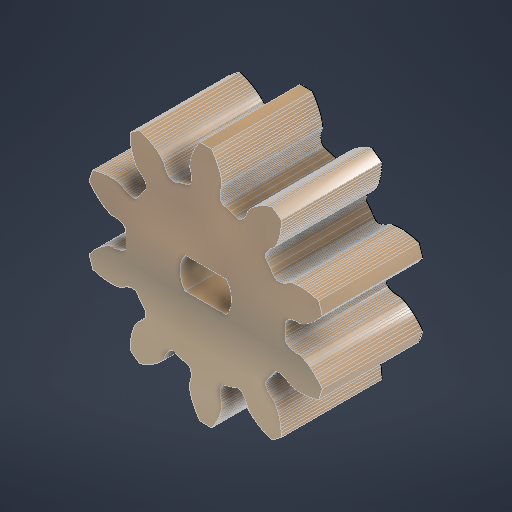
# Autodesk Inventor part: drive_gear_v1
Saved by Autodesk Inventor 2026.1 (Build 301233020, 233B)
## iProperties
Created: 2025-12-19
Part Number: drive_gear_v1
Material: Wood (Maple)
Document SubType Name: Modeling
Designer: colin
Density: 0.67 g/cm^3
Appearance: Natural Maple - Glossy Dark Tint
Autodesk Inventor part; units mm, degrees
(part 1 of 2)
ref_plane "YZ Plane" through (0, 0, 0) normal (1, 0, 0) x (0, 1, 0)
ref_plane "XZ Plane" through (0, 0, 0) normal (0, 1, 0) x (-1, 0, 0)
ref_plane "XY Plane" through (0, 0, 0) normal (0, 0, 1) x (1, 0, 0)
sketch "Sketch1" plane through (0, 0, 0) normal (0, 0, 1) x (1, 0, 0)
  point P0 (0, 0)
sketch "0" plane through (0, 0, 0) normal (0, 0, 1) x (1, 0, 0)
  line L0 (117.0437, 1.525) -> (112.9563, 1.525)
  line L1 (112.9563, -1.525) -> (117.0437, -1.525)
  line L2 (-25.3188, 0) -> (151.9129, 0) projected
  arc A0 (112.9563, 1.525) -> (112.9563, -1.525) centre (115, 0) ccw
  arc A1 (117.0437, -1.525) -> (117.0437, 1.525) centre (115, 0) ccw
  point P0 (119.0458, 0)
  point P1 (115.2341, -1.525)
  dimension "d8" = 3.05
  dimension "d9" = 2.55
  dimension "d10" = 2.55
  constraints: 4 end point, 4 point on circle, 2 centre point, 1 horizontal, 1 parallel, 1 point on line
  measures "d8" distance between parallel lines of L0 L1
  measures "d9" radius of A1
  measures "d10" radius of A0
sketch "layer0" plane through (0, 0, 0) normal (0, 0, 1) x (1, 0, 0)
  line L0 (107.4857, -9.0966) -> (107.5036, -8.8065)
  line L1 (107.5036, -8.8065) -> (107.532, -8.5336)
  line L2 (107.532, -8.5336) -> (107.5694, -8.2786)
  line L3 (107.5694, -8.2786) -> (107.6141, -8.0429)
  line L4 (107.6141, -8.0429) -> (107.6654, -7.8231)
  line L5 (107.6654, -7.8231) -> (107.721, -7.6228)
  line L6 (107.721, -7.6228) -> (107.7801, -7.4403)
  line L7 (107.7801, -7.4403) -> (107.8409, -7.2761)
  line L8 (107.8409, -7.2761) -> (107.9625, -7.0011)
  line L9 (107.9625, -7.0011) -> (108.0758, -6.7937)
  line L10 (108.0758, -6.7937) -> (108.1683, -6.6535)
  line L11 (108.1683, -6.6535) -> (108.218, -6.5889)
  line L12 (108.218, -6.5889) -> (108.3789, -6.4763)
  line L13 (108.3789, -6.4763) -> (108.5412, -6.345)
  line L14 (108.5412, -6.345) -> (108.681, -6.2122)
  line L15 (108.681, -6.2122) -> (108.7986, -6.0795)
  line L16 (108.7986, -6.0795) -> (108.8943, -5.9486)
  line L17 (108.8943, -5.9486) -> (108.9684, -5.821)
  line L18 (108.9684, -5.821) -> (109.0215, -5.6982)
  line L19 (109.0215, -5.6982) -> (109.054, -5.5819)
  line L20 (109.054, -5.5819) -> (109.0667, -5.4735)
  line L21 (109.0667, -5.4735) -> (109.0602, -5.3745)
  line L22 (109.0602, -5.3745) -> (109.0355, -5.2862)
  line L23 (109.0355, -5.2862) -> (108.987, -5.2014)
  line L24 (108.987, -5.2014) -> (108.8344, -5.0188)
  line L25 (108.8344, -5.0188) -> (108.5683, -4.6729)
  line L26 (108.5683, -4.6729) -> (108.3216, -4.313)
  line L27 (108.3216, -4.313) -> (108.1951, -4.1114)
  line L28 (108.1951, -4.1114) -> (108.1294, -4.0391)
  line L29 (108.1294, -4.0391) -> (108.0531, -3.9883)
  line L30 (108.0531, -3.9883) -> (107.9608, -3.9515)
  line L31 (107.9608, -3.9515) -> (107.8538, -3.9301)
  line L32 (107.8538, -3.9301) -> (107.7332, -3.9251)
  line L33 (107.7332, -3.9251) -> (107.6001, -3.9376)
  line L34 (107.6001, -3.9376) -> (107.4558, -3.9687)
  line L35 (107.4558, -3.9687) -> (107.3017, -4.0192)
  line L36 (107.3017, -4.0192) -> (107.1392, -4.0901)
  line L37 (107.1392, -4.0901) -> (106.9697, -4.182)
  line L38 (106.9697, -4.182) -> (106.7947, -4.2958)
  line L39 (106.7947, -4.2958) -> (106.6379, -4.414)
  line L40 (106.6379, -4.414) -> (106.561, -4.4413)
  line L41 (106.561, -4.4413) -> (106.3991, -4.4859)
  line L42 (106.3991, -4.4859) -> (106.1668, -4.5296)
  line L43 (106.1668, -4.5296) -> (105.8678, -4.5603)
  line L44 (105.8678, -4.5603) -> (105.6928, -4.5674)
  line L45 (105.6928, -4.5674) -> (105.5009, -4.5671)
  line L46 (105.5009, -4.5671) -> (105.2933, -4.5582)
  line L47 (105.2933, -4.5582) -> (105.0683, -4.539)
  line L48 (105.0683, -4.539) -> (104.8304, -4.5087)
  line L49 (104.8304, -4.5087) -> (104.5763, -4.4654)
  line L50 (104.5763, -4.4654) -> (104.308, -4.4081)
  line L51 (104.308, -4.4081) -> (104.0266, -4.3355)
  line L52 (104.0266, -4.3355) -> (103.7825, -4.2622)
  arc A0 (103.4196, -3.1453) -> (103.7825, -4.2622) centre (115.0001, 0) ccw
  line L53 (103.4196, -3.1453) -> (103.574, -2.9425)
  line L54 (103.574, -2.9425) -> (103.759, -2.7184)
  line L55 (103.759, -2.7184) -> (103.9423, -2.5143)
  line L56 (103.9423, -2.5143) -> (104.1225, -2.33)
  line L57 (104.1225, -2.33) -> (104.2971, -2.1655)
  line L58 (104.2971, -2.1655) -> (104.4678, -2.0178)
  line L59 (104.4678, -2.0178) -> (104.6306, -1.8885)
  line L60 (104.6306, -1.8885) -> (104.7857, -1.7756)
  line L61 (104.7857, -1.7756) -> (104.9314, -1.6785)
  line L62 (104.9314, -1.6785) -> (105.1914, -1.5275)
  line L63 (105.1914, -1.5275) -> (105.405, -1.4263)
  line L64 (105.405, -1.4263) -> (105.5622, -1.3672)
  line L65 (105.5622, -1.3672) -> (105.6405, -1.3442)
  line L66 (105.6405, -1.3442) -> (105.8368, -1.3476)
  line L67 (105.8368, -1.3476) -> (106.0452, -1.3368)
  line L68 (106.0452, -1.3368) -> (106.2364, -1.3115)
  line L69 (106.2364, -1.3115) -> (106.4095, -1.2733)
  line L70 (106.4095, -1.2733) -> (106.5639, -1.2237)
  line L71 (106.5639, -1.2237) -> (106.6989, -1.164)
  line L72 (106.6989, -1.164) -> (106.8139, -1.0959)
  line L73 (106.8139, -1.0959) -> (106.9086, -1.0209)
  line L74 (106.9086, -1.0209) -> (106.9826, -0.9407)
  line L75 (106.9826, -0.9407) -> (107.0356, -0.8567)
  line L76 (107.0356, -0.8567) -> (107.0675, -0.7708)
  line L77 (107.0675, -0.7708) -> (107.0781, -0.6736)
  line L78 (107.0781, -0.6736) -> (107.062, -0.4362)
  line L79 (107.062, -0.4362) -> (107.05, 0)
  line L80 (107.05, 0) -> (107.062, 0.4362)
  line L81 (107.062, 0.4362) -> (107.0781, 0.6736)
  line L82 (107.0781, 0.6736) -> (107.0675, 0.7708)
  line L83 (107.0675, 0.7708) -> (107.0356, 0.8567)
  line L84 (107.0356, 0.8567) -> (106.9826, 0.9407)
  line L85 (106.9826, 0.9407) -> (106.9086, 1.0209)
  line L86 (106.9086, 1.0209) -> (106.8139, 1.0959)
  line L87 (106.8139, 1.0959) -> (106.6989, 1.164)
  line L88 (106.6989, 1.164) -> (106.5639, 1.2237)
  line L89 (106.5639, 1.2237) -> (106.4095, 1.2733)
  line L90 (106.4095, 1.2733) -> (106.2364, 1.3115)
  line L91 (106.2364, 1.3115) -> (106.0452, 1.3368)
  line L92 (106.0452, 1.3368) -> (105.8368, 1.3476)
  line L93 (105.8368, 1.3476) -> (105.6405, 1.3442)
  line L94 (105.6405, 1.3442) -> (105.5622, 1.3672)
  line L95 (105.5622, 1.3672) -> (105.405, 1.4263)
  line L96 (105.405, 1.4263) -> (105.1914, 1.5275)
  line L97 (105.1914, 1.5275) -> (104.9314, 1.6785)
  line L98 (104.9314, 1.6785) -> (104.7857, 1.7756)
  line L99 (104.7857, 1.7756) -> (104.6306, 1.8885)
  line L100 (104.6306, 1.8885) -> (104.4678, 2.0178)
  line L101 (104.4678, 2.0178) -> (104.2971, 2.1655)
  line L102 (104.2971, 2.1655) -> (104.1225, 2.33)
  line L103 (104.1225, 2.33) -> (103.9423, 2.5143)
  line L104 (103.9423, 2.5143) -> (103.759, 2.7184)
  line L105 (103.759, 2.7184) -> (103.574, 2.9425)
  line L106 (103.574, 2.9425) -> (103.4196, 3.1453)
  arc A1 (103.7825, 4.2622) -> (103.4196, 3.1453) centre (115.0001, 0) ccw
  line L107 (103.7825, 4.2622) -> (104.0266, 4.3355)
  line L108 (104.0266, 4.3355) -> (104.308, 4.4081)
  line L109 (104.308, 4.4081) -> (104.5763, 4.4654)
  line L110 (104.5763, 4.4654) -> (104.8304, 4.5087)
  line L111 (104.8304, 4.5087) -> (105.0683, 4.539)
  line L112 (105.0683, 4.539) -> (105.2933, 4.5582)
  line L113 (105.2933, 4.5582) -> (105.5009, 4.5671)
  line L114 (105.5009, 4.5671) -> (105.6928, 4.5674)
  line L115 (105.6928, 4.5674) -> (105.8678, 4.5603)
  line L116 (105.8678, 4.5603) -> (106.1668, 4.5296)
  line L117 (106.1668, 4.5296) -> (106.3991, 4.4859)
  line L118 (106.3991, 4.4859) -> (106.561, 4.4413)
  line L119 (106.561, 4.4413) -> (106.6379, 4.414)
  line L120 (106.6379, 4.414) -> (106.7947, 4.2958)
  line L121 (106.7947, 4.2958) -> (106.9697, 4.182)
  line L122 (106.9697, 4.182) -> (107.1392, 4.0901)
  line L123 (107.1392, 4.0901) -> (107.3017, 4.0192)
  line L124 (107.3017, 4.0192) -> (107.4558, 3.9687)
  line L125 (107.4558, 3.9687) -> (107.6001, 3.9376)
  line L126 (107.6001, 3.9376) -> (107.7332, 3.9251)
  line L127 (107.7332, 3.9251) -> (107.8538, 3.9301)
  line L128 (107.8538, 3.9301) -> (107.9608, 3.9515)
  line L129 (107.9608, 3.9515) -> (108.0531, 3.9883)
  line L130 (108.0531, 3.9883) -> (108.1294, 4.0391)
  line L131 (108.1294, 4.0391) -> (108.1951, 4.1114)
  line L132 (108.1951, 4.1114) -> (108.3216, 4.313)
  line L133 (108.3216, 4.313) -> (108.5683, 4.6729)
  line L134 (108.5683, 4.6729) -> (108.8344, 5.0188)
  line L135 (108.8344, 5.0188) -> (108.987, 5.2014)
  line L136 (108.987, 5.2014) -> (109.0355, 5.2862)
  line L137 (109.0355, 5.2862) -> (109.0602, 5.3745)
  line L138 (109.0602, 5.3745) -> (109.0667, 5.4735)
  line L139 (109.0667, 5.4735) -> (109.054, 5.5819)
  line L140 (109.054, 5.5819) -> (109.0215, 5.6982)
  line L141 (109.0215, 5.6982) -> (108.9684, 5.821)
  line L142 (108.9684, 5.821) -> (108.8943, 5.9486)
  line L143 (108.8943, 5.9486) -> (108.7986, 6.0795)
  line L144 (108.7986, 6.0795) -> (108.681, 6.2122)
  line L145 (108.681, 6.2122) -> (108.5412, 6.345)
  line L146 (108.5412, 6.345) -> (108.3789, 6.4763)
  line L147 (108.3789, 6.4763) -> (108.218, 6.5889)
  line L148 (108.218, 6.5889) -> (108.1683, 6.6535)
  line L149 (108.1683, 6.6535) -> (108.0758, 6.7937)
  line L150 (108.0758, 6.7937) -> (107.9625, 7.0011)
  line L151 (107.9625, 7.0011) -> (107.8409, 7.2761)
  line L152 (107.8409, 7.2761) -> (107.7801, 7.4403)
  line L153 (107.7801, 7.4403) -> (107.721, 7.6228)
  line L154 (107.721, 7.6228) -> (107.6654, 7.8231)
  line L155 (107.6654, 7.8231) -> (107.6141, 8.0429)
  line L156 (107.6141, 8.0429) -> (107.5694, 8.2786)
  line L157 (107.5694, 8.2786) -> (107.532, 8.5336)
  line L158 (107.532, 8.5336) -> (107.5036, 8.8065)
  line L159 (107.5036, 8.8065) -> (107.4857, 9.0966)
  line L160 (107.4857, 9.0966) -> (107.48, 9.3514)
  arc A2 (108.4301, 10.0416) -> (107.48, 9.3514) centre (115, -0.0001) ccw
  line L161 (108.4301, 10.0416) -> (108.6707, 9.9575)
  line L162 (108.6707, 9.9575) -> (108.941, 9.8508)
  line L163 (108.941, 9.8508) -> (109.1918, 9.7395)
  line L164 (109.1918, 9.7395) -> (109.4227, 9.6252)
  line L165 (109.4227, 9.6252) -> (109.6331, 9.5098)
  line L166 (109.6331, 9.5098) -> (109.8263, 9.3931)
  line L167 (109.8263, 9.3931) -> (109.9996, 9.2783)
  line L168 (109.9996, 9.2783) -> (110.155, 9.1657)
  line L169 (110.155, 9.1657) -> (110.2923, 9.0571)
  line L170 (110.2923, 9.0571) -> (110.5162, 8.8565)
  line L171 (110.5162, 8.8565) -> (110.6785, 8.6847)
  line L172 (110.6785, 8.6847) -> (110.7833, 8.5534)
  line L173 (110.7833, 8.5534) -> (110.8294, 8.4861)
  line L174 (110.8294, 8.4861) -> (110.8867, 8.2983)
  line L175 (110.8867, 8.2983) -> (110.9615, 8.1034)
  line L176 (110.9615, 8.1034) -> (111.0445, 7.9294)
  line L177 (111.0445, 7.9294) -> (111.1344, 7.7765)
  line L178 (111.1344, 7.7765) -> (111.2293, 7.6451)
  line L179 (111.2293, 7.6451) -> (111.3278, 7.5351)
  line L180 (111.3278, 7.5351) -> (111.4281, 7.4468)
  line L181 (111.4281, 7.4468) -> (111.5287, 7.3799)
  line L182 (111.5287, 7.3799) -> (111.6279, 7.3344)
  line L183 (111.6279, 7.3344) -> (111.724, 7.3099)
  line L184 (111.724, 7.3099) -> (111.8157, 7.3061)
  line L185 (111.8157, 7.3061) -> (111.9113, 7.3261)
  line L186 (111.9113, 7.3261) -> (112.1321, 7.4147)
  line L187 (112.1321, 7.4147) -> (112.5433, 7.5609)
  line L188 (112.5433, 7.5609) -> (112.9619, 7.6843)
  line L189 (112.9619, 7.6843) -> (113.1926, 7.7424)
  line L190 (113.1926, 7.7424) -> (113.2818, 7.7825)
  line L191 (113.2818, 7.7825) -> (113.3537, 7.8394)
  line L192 (113.3537, 7.8394) -> (113.4171, 7.9157)
  line L193 (113.4171, 7.9157) -> (113.4706, 8.0109)
  line L194 (113.4706, 8.0109) -> (113.5126, 8.1241)
  line L195 (113.5126, 8.1241) -> (113.5418, 8.2545)
  line L196 (113.5418, 8.2545) -> (113.5569, 8.4013)
  line L197 (113.5569, 8.4013) -> (113.5564, 8.5635)
  line L198 (113.5564, 8.5635) -> (113.5393, 8.74)
  line L199 (113.5393, 8.74) -> (113.5042, 8.9296)
  line L200 (113.5042, 8.9296) -> (113.4501, 9.1312)
  line L201 (113.4501, 9.1312) -> (113.3861, 9.3168)
  line L202 (113.3861, 9.3168) -> (113.3839, 9.3984)
  line L203 (113.3839, 9.3984) -> (113.3915, 9.5662)
  line L204 (113.3915, 9.5662) -> (113.4217, 9.8006)
  line L205 (113.4217, 9.8006) -> (113.485, 10.0945)
  line L206 (113.485, 10.0945) -> (113.5322, 10.2631)
  line L207 (113.5322, 10.2631) -> (113.5918, 10.4455)
  line L208 (113.5918, 10.4455) -> (113.6644, 10.6402)
  line L209 (113.6644, 10.6402) -> (113.7522, 10.8482)
  line L210 (113.7522, 10.8482) -> (113.8546, 11.0652)
  line L211 (113.8546, 11.0652) -> (113.9742, 11.2934)
  line L212 (113.9742, 11.2934) -> (114.1116, 11.5309)
  line L213 (114.1116, 11.5309) -> (114.2676, 11.7761)
  line L214 (114.2676, 11.7761) -> (114.4128, 11.9856)
  arc A3 (115.5872, 11.9856) -> (114.4128, 11.9856) centre (115, -0.0001) ccw
  line L215 (115.5872, 11.9856) -> (115.7324, 11.7761)
  line L216 (115.7324, 11.7761) -> (115.8884, 11.5309)
  line L217 (115.8884, 11.5309) -> (116.0258, 11.2934)
  line L218 (116.0258, 11.2934) -> (116.1454, 11.0652)
  line L219 (116.1454, 11.0652) -> (116.2478, 10.8482)
  line L220 (116.2478, 10.8482) -> (116.3356, 10.6402)
  line L221 (116.3356, 10.6402) -> (116.4082, 10.4455)
  line L222 (116.4082, 10.4455) -> (116.4678, 10.2631)
  line L223 (116.4678, 10.2631) -> (116.515, 10.0945)
  line L224 (116.515, 10.0945) -> (116.5783, 9.8006)
  line L225 (116.5783, 9.8006) -> (116.6085, 9.5662)
  line L226 (116.6085, 9.5662) -> (116.6161, 9.3984)
  line L227 (116.6161, 9.3984) -> (116.6139, 9.3168)
  line L228 (116.6139, 9.3168) -> (116.5499, 9.1312)
  line L229 (116.5499, 9.1312) -> (116.4958, 8.9296)
  line L230 (116.4958, 8.9296) -> (116.4607, 8.74)
  line L231 (116.4607, 8.74) -> (116.4436, 8.5635)
  line L232 (116.4436, 8.5635) -> (116.4431, 8.4013)
  line L233 (116.4431, 8.4013) -> (116.4582, 8.2545)
  line L234 (116.4582, 8.2545) -> (116.4874, 8.1241)
  line L235 (116.4874, 8.1241) -> (116.5294, 8.0109)
  line L236 (116.5294, 8.0109) -> (116.5829, 7.9157)
  line L237 (116.5829, 7.9157) -> (116.6463, 7.8394)
  line L238 (116.6463, 7.8394) -> (116.7182, 7.7825)
  line L239 (116.7182, 7.7825) -> (116.8074, 7.7424)
  line L240 (116.8074, 7.7424) -> (117.0381, 7.6843)
  line L241 (117.0381, 7.6843) -> (117.4567, 7.5609)
  line L242 (117.4567, 7.5609) -> (117.8679, 7.4147)
  line L243 (117.8679, 7.4147) -> (118.0887, 7.3261)
  line L244 (118.0887, 7.3261) -> (118.1843, 7.3061)
  line L245 (118.1843, 7.3061) -> (118.276, 7.3099)
  line L246 (118.276, 7.3099) -> (118.3721, 7.3344)
  line L247 (118.3721, 7.3344) -> (118.4713, 7.3799)
  line L248 (118.4713, 7.3799) -> (118.5719, 7.4468)
  line L249 (118.5719, 7.4468) -> (118.6722, 7.5351)
  line L250 (118.6722, 7.5351) -> (118.7707, 7.6451)
  line L251 (118.7707, 7.6451) -> (118.8656, 7.7765)
  line L252 (118.8656, 7.7765) -> (118.9555, 7.9294)
  line L253 (118.9555, 7.9294) -> (119.0385, 8.1034)
  line L254 (119.0385, 8.1034) -> (119.1133, 8.2983)
  line L255 (119.1133, 8.2983) -> (119.1706, 8.4861)
  line L256 (119.1706, 8.4861) -> (119.2167, 8.5534)
  line L257 (119.2167, 8.5534) -> (119.3215, 8.6847)
  line L258 (119.3215, 8.6847) -> (119.4838, 8.8565)
  line L259 (119.4838, 8.8565) -> (119.7077, 9.0571)
  line L260 (119.7077, 9.0571) -> (119.845, 9.1657)
  line L261 (119.845, 9.1657) -> (120.0004, 9.2783)
  line L262 (120.0004, 9.2783) -> (120.1737, 9.3931)
  line L263 (120.1737, 9.3931) -> (120.3669, 9.5098)
  line L264 (120.3669, 9.5098) -> (120.5773, 9.6252)
  line L265 (120.5773, 9.6252) -> (120.8082, 9.7395)
  line L266 (120.8082, 9.7395) -> (121.059, 9.8508)
  line L267 (121.059, 9.8508) -> (121.3293, 9.9575)
  line L268 (121.3293, 9.9575) -> (121.5699, 10.0416)
  arc A4 (122.52, 9.3514) -> (121.5699, 10.0416) centre (115, -0.0001) ccw
  line L269 (122.52, 9.3514) -> (122.5143, 9.0966)
  line L270 (122.5143, 9.0966) -> (122.4964, 8.8065)
  line L271 (122.4964, 8.8065) -> (122.468, 8.5336)
  line L272 (122.468, 8.5336) -> (122.4306, 8.2786)
  line L273 (122.4306, 8.2786) -> (122.3859, 8.0429)
  line L274 (122.3859, 8.0429) -> (122.3346, 7.8231)
  line L275 (122.3346, 7.8231) -> (122.279, 7.6228)
  line L276 (122.279, 7.6228) -> (122.2199, 7.4403)
  line L277 (122.2199, 7.4403) -> (122.1591, 7.2761)
  line L278 (122.1591, 7.2761) -> (122.0375, 7.0011)
  line L279 (122.0375, 7.0011) -> (121.9242, 6.7937)
  line L280 (121.9242, 6.7937) -> (121.8317, 6.6535)
  line L281 (121.8317, 6.6535) -> (121.782, 6.5889)
  line L282 (121.782, 6.5889) -> (121.6211, 6.4763)
  line L283 (121.6211, 6.4763) -> (121.4588, 6.345)
  line L284 (121.4588, 6.345) -> (121.319, 6.2122)
  line L285 (121.319, 6.2122) -> (121.2014, 6.0795)
  line L286 (121.2014, 6.0795) -> (121.1057, 5.9486)
  line L287 (121.1057, 5.9486) -> (121.0316, 5.821)
  line L288 (121.0316, 5.821) -> (120.9785, 5.6982)
  line L289 (120.9785, 5.6982) -> (120.946, 5.5819)
  line L290 (120.946, 5.5819) -> (120.9333, 5.4735)
  line L291 (120.9333, 5.4735) -> (120.9398, 5.3745)
  line L292 (120.9398, 5.3745) -> (120.9645, 5.2862)
  line L293 (120.9645, 5.2862) -> (121.013, 5.2014)
  line L294 (121.013, 5.2014) -> (121.1656, 5.0188)
  line L295 (121.1656, 5.0188) -> (121.4317, 4.6729)
  line L296 (121.4317, 4.6729) -> (121.6784, 4.313)
  line L297 (121.6784, 4.313) -> (121.8049, 4.1114)
  line L298 (121.8049, 4.1114) -> (121.8706, 4.0391)
  line L299 (121.8706, 4.0391) -> (121.9469, 3.9883)
  line L300 (121.9469, 3.9883) -> (122.0392, 3.9515)
  line L301 (122.0392, 3.9515) -> (122.1462, 3.9301)
  line L302 (122.1462, 3.9301) -> (122.2668, 3.9251)
  line L303 (122.2668, 3.9251) -> (122.3999, 3.9376)
  line L304 (122.3999, 3.9376) -> (122.5442, 3.9687)
  line L305 (122.5442, 3.9687) -> (122.6983, 4.0192)
  line L306 (122.6983, 4.0192) -> (122.8608, 4.0901)
  line L307 (122.8608, 4.0901) -> (123.0303, 4.182)
  line L308 (123.0303, 4.182) -> (123.2053, 4.2958)
  line L309 (123.2053, 4.2958) -> (123.3621, 4.414)
  line L310 (123.3621, 4.414) -> (123.439, 4.4413)
  line L311 (123.439, 4.4413) -> (123.6009, 4.4859)
  line L312 (123.6009, 4.4859) -> (123.8332, 4.5296)
  line L313 (123.8332, 4.5296) -> (124.1322, 4.5603)
  line L314 (124.1322, 4.5603) -> (124.3072, 4.5674)
  line L315 (124.3072, 4.5674) -> (124.4991, 4.5671)
  line L316 (124.4991, 4.5671) -> (124.7067, 4.5582)
  line L317 (124.7067, 4.5582) -> (124.9317, 4.539)
  line L318 (124.9317, 4.539) -> (125.1696, 4.5087)
  line L319 (125.1696, 4.5087) -> (125.4237, 4.4654)
  line L320 (125.4237, 4.4654) -> (125.692, 4.4081)
  line L321 (125.692, 4.4081) -> (125.9734, 4.3355)
  line L322 (125.9734, 4.3355) -> (126.2175, 4.2622)
  arc A5 (126.5804, 3.1453) -> (126.2175, 4.2622) centre (114.9999, 0) ccw
  line L323 (126.5804, 3.1453) -> (126.426, 2.9425)
  line L324 (126.426, 2.9425) -> (126.241, 2.7184)
  line L325 (126.241, 2.7184) -> (126.0577, 2.5143)
  line L326 (126.0577, 2.5143) -> (125.8775, 2.33)
  line L327 (125.8775, 2.33) -> (125.7029, 2.1655)
  line L328 (125.7029, 2.1655) -> (125.5322, 2.0178)
  line L329 (125.5322, 2.0178) -> (125.3694, 1.8885)
  line L330 (125.3694, 1.8885) -> (125.2143, 1.7756)
  line L331 (125.2143, 1.7756) -> (125.0686, 1.6785)
  line L332 (125.0686, 1.6785) -> (124.8086, 1.5275)
  line L333 (124.8086, 1.5275) -> (124.595, 1.4263)
  line L334 (124.595, 1.4263) -> (124.4378, 1.3672)
  line L335 (124.4378, 1.3672) -> (124.3595, 1.3442)
  line L336 (124.3595, 1.3442) -> (124.1632, 1.3476)
  line L337 (124.1632, 1.3476) -> (123.9548, 1.3368)
  line L338 (123.9548, 1.3368) -> (123.7636, 1.3115)
  line L339 (123.7636, 1.3115) -> (123.5905, 1.2733)
  line L340 (123.5905, 1.2733) -> (123.4361, 1.2237)
  line L341 (123.4361, 1.2237) -> (123.3011, 1.164)
  line L342 (123.3011, 1.164) -> (123.1861, 1.0959)
  line L343 (123.1861, 1.0959) -> (123.0914, 1.0209)
  line L344 (123.0914, 1.0209) -> (123.0174, 0.9407)
  line L345 (123.0174, 0.9407) -> (122.9644, 0.8567)
  line L346 (122.9644, 0.8567) -> (122.9325, 0.7708)
  line L347 (122.9325, 0.7708) -> (122.9219, 0.6736)
  line L348 (122.9219, 0.6736) -> (122.9381, 0.4362)
  line L349 (122.9381, 0.4362) -> (122.95, 0)
  line L350 (122.95, 0) -> (122.9381, -0.4362)
  line L351 (122.9381, -0.4362) -> (122.9219, -0.6736)
  line L352 (122.9219, -0.6736) -> (122.9325, -0.7708)
  line L353 (122.9325, -0.7708) -> (122.9644, -0.8567)
  line L354 (122.9644, -0.8567) -> (123.0174, -0.9407)
  line L355 (123.0174, -0.9407) -> (123.0914, -1.0209)
  line L356 (123.0914, -1.0209) -> (123.1861, -1.0959)
  line L357 (123.1861, -1.0959) -> (123.3011, -1.164)
  line L358 (123.3011, -1.164) -> (123.4361, -1.2237)
  line L359 (123.4361, -1.2237) -> (123.5905, -1.2733)
  line L360 (123.5905, -1.2733) -> (123.7636, -1.3115)
  line L361 (123.7636, -1.3115) -> (123.9548, -1.3368)
  line L362 (123.9548, -1.3368) -> (124.1632, -1.3476)
  line L363 (124.1632, -1.3476) -> (124.3595, -1.3442)
  line L364 (124.3595, -1.3442) -> (124.4378, -1.3672)
  line L365 (124.4378, -1.3672) -> (124.595, -1.4263)
  line L366 (124.595, -1.4263) -> (124.8086, -1.5275)
  line L367 (124.8086, -1.5275) -> (125.0686, -1.6785)
  line L368 (125.0686, -1.6785) -> (125.2143, -1.7756)
  line L369 (125.2143, -1.7756) -> (125.3694, -1.8885)
  line L370 (125.3694, -1.8885) -> (125.5322, -2.0178)
  line L371 (125.5322, -2.0178) -> (125.7029, -2.1655)
  line L372 (125.7029, -2.1655) -> (125.8775, -2.33)
  line L373 (125.8775, -2.33) -> (126.0577, -2.5143)
  line L374 (126.0577, -2.5143) -> (126.241, -2.7184)
  line L375 (126.241, -2.7184) -> (126.426, -2.9425)
  line L376 (126.426, -2.9425) -> (126.5804, -3.1453)
  arc A6 (126.2175, -4.2622) -> (126.5804, -3.1453) centre (114.9999, 0) ccw
  line L377 (126.2175, -4.2622) -> (125.9734, -4.3355)
  line L378 (125.9734, -4.3355) -> (125.692, -4.4081)
  line L379 (125.692, -4.4081) -> (125.4237, -4.4654)
  line L380 (125.4237, -4.4654) -> (125.1696, -4.5087)
  line L381 (125.1696, -4.5087) -> (124.9317, -4.539)
  line L382 (124.9317, -4.539) -> (124.7067, -4.5582)
  line L383 (124.7067, -4.5582) -> (124.4991, -4.5671)
  line L384 (124.4991, -4.5671) -> (124.3072, -4.5674)
  line L385 (124.3072, -4.5674) -> (124.1322, -4.5603)
  line L386 (124.1322, -4.5603) -> (123.8332, -4.5296)
  line L387 (123.8332, -4.5296) -> (123.6009, -4.4859)
  line L388 (123.6009, -4.4859) -> (123.439, -4.4413)
  line L389 (123.439, -4.4413) -> (123.3621, -4.414)
  line L390 (123.3621, -4.414) -> (123.2053, -4.2958)
  line L391 (123.2053, -4.2958) -> (123.0303, -4.182)
  line L392 (123.0303, -4.182) -> (122.8608, -4.0901)
  line L393 (122.8608, -4.0901) -> (122.6983, -4.0192)
  line L394 (122.6983, -4.0192) -> (122.5442, -3.9687)
  line L395 (122.5442, -3.9687) -> (122.3999, -3.9376)
  line L396 (122.3999, -3.9376) -> (122.2668, -3.9251)
  line L397 (122.2668, -3.9251) -> (122.1462, -3.9301)
  line L398 (122.1462, -3.9301) -> (122.0392, -3.9515)
  line L399 (122.0392, -3.9515) -> (121.9469, -3.9883)
  line L400 (121.9469, -3.9883) -> (121.8706, -4.0391)
  line L401 (121.8706, -4.0391) -> (121.8049, -4.1114)
  line L402 (121.8049, -4.1114) -> (121.6784, -4.313)
  line L403 (121.6784, -4.313) -> (121.4317, -4.6729)
  line L404 (121.4317, -4.6729) -> (121.1656, -5.0188)
  line L405 (121.1656, -5.0188) -> (121.013, -5.2014)
  line L406 (121.013, -5.2014) -> (120.9645, -5.2862)
  line L407 (120.9645, -5.2862) -> (120.9398, -5.3745)
  line L408 (120.9398, -5.3745) -> (120.9333, -5.4735)
  line L409 (120.9333, -5.4735) -> (120.946, -5.5819)
  line L410 (120.946, -5.5819) -> (120.9785, -5.6982)
  line L411 (120.9785, -5.6982) -> (121.0316, -5.821)
  line L412 (121.0316, -5.821) -> (121.1057, -5.9486)
  line L413 (121.1057, -5.9486) -> (121.2014, -6.0795)
  line L414 (121.2014, -6.0795) -> (121.319, -6.2122)
  line L415 (121.319, -6.2122) -> (121.4588, -6.345)
  line L416 (121.4588, -6.345) -> (121.6211, -6.4763)
  line L417 (121.6211, -6.4763) -> (121.782, -6.5889)
  line L418 (121.782, -6.5889) -> (121.8317, -6.6535)
  line L419 (121.8317, -6.6535) -> (121.9242, -6.7937)
  line L420 (121.9242, -6.7937) -> (122.0375, -7.0011)
  line L421 (122.0375, -7.0011) -> (122.1591, -7.2761)
  line L422 (122.1591, -7.2761) -> (122.2199, -7.4403)
  line L423 (122.2199, -7.4403) -> (122.279, -7.6228)
  line L424 (122.279, -7.6228) -> (122.3346, -7.8231)
  line L425 (122.3346, -7.8231) -> (122.3859, -8.0429)
  line L426 (122.3859, -8.0429) -> (122.4306, -8.2786)
  line L427 (122.4306, -8.2786) -> (122.468, -8.5336)
  line L428 (122.468, -8.5336) -> (122.4964, -8.8065)
  line L429 (122.4964, -8.8065) -> (122.5143, -9.0966)
  line L430 (122.5143, -9.0966) -> (122.52, -9.3514)
  arc A7 (121.5699, -10.0416) -> (122.52, -9.3514) centre (115, 0.0001) ccw
  line L431 (121.5699, -10.0416) -> (121.3293, -9.9575)
  line L432 (121.3293, -9.9575) -> (121.059, -9.8508)
  line L433 (121.059, -9.8508) -> (120.8082, -9.7395)
  line L434 (120.8082, -9.7395) -> (120.5773, -9.6252)
  line L435 (120.5773, -9.6252) -> (120.3669, -9.5098)
  line L436 (120.3669, -9.5098) -> (120.1737, -9.3931)
  line L437 (120.1737, -9.3931) -> (120.0004, -9.2783)
  line L438 (120.0004, -9.2783) -> (119.845, -9.1657)
  line L439 (119.845, -9.1657) -> (119.7077, -9.0571)
  line L440 (119.7077, -9.0571) -> (119.4838, -8.8565)
  line L441 (119.4838, -8.8565) -> (119.3215, -8.6847)
  line L442 (119.3215, -8.6847) -> (119.2167, -8.5534)
  line L443 (119.2167, -8.5534) -> (119.1706, -8.4861)
  line L444 (119.1706, -8.4861) -> (119.1133, -8.2983)
  line L445 (119.1133, -8.2983) -> (119.0385, -8.1034)
  line L446 (119.0385, -8.1034) -> (118.9555, -7.9294)
  line L447 (118.9555, -7.9294) -> (118.8656, -7.7765)
  line L448 (118.8656, -7.7765) -> (118.7707, -7.6451)
  line L449 (118.7707, -7.6451) -> (118.6722, -7.5351)
  line L450 (118.6722, -7.5351) -> (118.5719, -7.4468)
  line L451 (118.5719, -7.4468) -> (118.4713, -7.3799)
  line L452 (118.4713, -7.3799) -> (118.3721, -7.3344)
  line L453 (118.3721, -7.3344) -> (118.276, -7.3099)
  line L454 (118.276, -7.3099) -> (118.1843, -7.3061)
  line L455 (118.1843, -7.3061) -> (118.0887, -7.3261)
  line L456 (118.0887, -7.3261) -> (117.8679, -7.4147)
  line L457 (117.8679, -7.4147) -> (117.4567, -7.5609)
  line L458 (117.4567, -7.5609) -> (117.0381, -7.6843)
  line L459 (117.0381, -7.6843) -> (116.8074, -7.7424)
  line L460 (116.8074, -7.7424) -> (116.7182, -7.7825)
  line L461 (116.7182, -7.7825) -> (116.6463, -7.8394)
  line L462 (116.6463, -7.8394) -> (116.5829, -7.9157)
  line L463 (116.5829, -7.9157) -> (116.5294, -8.0109)
  line L464 (116.5294, -8.0109) -> (116.4874, -8.1241)
  line L465 (116.4874, -8.1241) -> (116.4582, -8.2545)
  line L466 (116.4582, -8.2545) -> (116.4431, -8.4013)
  line L467 (116.4431, -8.4013) -> (116.4436, -8.5635)
  line L468 (116.4436, -8.5635) -> (116.4607, -8.74)
  line L469 (116.4607, -8.74) -> (116.4958, -8.9296)
  line L470 (116.4958, -8.9296) -> (116.5499, -9.1312)
  line L471 (116.5499, -9.1312) -> (116.6139, -9.3168)
  line L472 (116.6139, -9.3168) -> (116.6161, -9.3984)
  line L473 (116.6161, -9.3984) -> (116.6085, -9.5662)
  line L474 (116.6085, -9.5662) -> (116.5783, -9.8006)
  line L475 (116.5783, -9.8006) -> (116.515, -10.0945)
  line L476 (116.515, -10.0945) -> (116.4678, -10.2631)
  line L477 (116.4678, -10.2631) -> (116.4082, -10.4455)
  line L478 (116.4082, -10.4455) -> (116.3356, -10.6402)
  line L479 (116.3356, -10.6402) -> (116.2478, -10.8482)
  line L480 (116.2478, -10.8482) -> (116.1454, -11.0652)
  line L481 (116.1454, -11.0652) -> (116.0258, -11.2934)
  line L482 (116.0258, -11.2934) -> (115.8884, -11.5309)
  line L483 (115.8884, -11.5309) -> (115.7324, -11.7761)
  line L484 (115.7324, -11.7761) -> (115.5872, -11.9856)
  arc A8 (114.4128, -11.9856) -> (115.5872, -11.9856) centre (115, 0.0001) ccw
  line L485 (114.4128, -11.9856) -> (114.2676, -11.7761)
  line L486 (114.2676, -11.7761) -> (114.1116, -11.5309)
  line L487 (114.1116, -11.5309) -> (113.9742, -11.2934)
  line L488 (113.9742, -11.2934) -> (113.8546, -11.0652)
  line L489 (113.8546, -11.0652) -> (113.7522, -10.8482)
  line L490 (113.7522, -10.8482) -> (113.6644, -10.6402)
  line L491 (113.6644, -10.6402) -> (113.5918, -10.4455)
  line L492 (113.5918, -10.4455) -> (113.5322, -10.2631)
  line L493 (113.5322, -10.2631) -> (113.485, -10.0945)
  line L494 (113.485, -10.0945) -> (113.4217, -9.8006)
  line L495 (113.4217, -9.8006) -> (113.3915, -9.5662)
  line L496 (113.3915, -9.5662) -> (113.3839, -9.3984)
  line L497 (113.3839, -9.3984) -> (113.3861, -9.3168)
  line L498 (113.3861, -9.3168) -> (113.4501, -9.1312)
  line L499 (113.4501, -9.1312) -> (113.5042, -8.9296)
  line L500 (113.5042, -8.9296) -> (113.5393, -8.74)
  line L501 (113.5393, -8.74) -> (113.5564, -8.5635)
  line L502 (113.5564, -8.5635) -> (113.5569, -8.4013)
  line L503 (113.5569, -8.4013) -> (113.5418, -8.2545)
  line L504 (113.5418, -8.2545) -> (113.5126, -8.1241)
  line L505 (113.5126, -8.1241) -> (113.4706, -8.0109)
  line L506 (113.4706, -8.0109) -> (113.4171, -7.9157)
  line L507 (113.4171, -7.9157) -> (113.3537, -7.8394)
  line L508 (113.3537, -7.8394) -> (113.2818, -7.7825)
  line L509 (113.2818, -7.7825) -> (113.1926, -7.7424)
  line L510 (113.1926, -7.7424) -> (112.9619, -7.6843)
  line L511 (112.9619, -7.6843) -> (112.5433, -7.5609)
  line L512 (112.5433, -7.5609) -> (112.1321, -7.4147)
  line L513 (112.1321, -7.4147) -> (111.9113, -7.3261)
  line L514 (111.9113, -7.3261) -> (111.8157, -7.3061)
  line L515 (111.8157, -7.3061) -> (111.724, -7.3099)
  line L516 (111.724, -7.3099) -> (111.6279, -7.3344)
  line L517 (111.6279, -7.3344) -> (111.5287, -7.3799)
  line L518 (111.5287, -7.3799) -> (111.4281, -7.4468)
  line L519 (111.4281, -7.4468) -> (111.3278, -7.5351)
  line L520 (111.3278, -7.5351) -> (111.2293, -7.6451)
  line L521 (111.2293, -7.6451) -> (111.1344, -7.7765)
  line L522 (111.1344, -7.7765) -> (111.0445, -7.9294)
  line L523 (111.0445, -7.9294) -> (110.9615, -8.1034)
  line L524 (110.9615, -8.1034) -> (110.8867, -8.2983)
  line L525 (110.8867, -8.2983) -> (110.8294, -8.4861)
  line L526 (110.8294, -8.4861) -> (110.7833, -8.5534)
  line L527 (110.7833, -8.5534) -> (110.6785, -8.6847)
  line L528 (110.6785, -8.6847) -> (110.5162, -8.8565)
  line L529 (110.5162, -8.8565) -> (110.2923, -9.0571)
  line L530 (110.2923, -9.0571) -> (110.155, -9.1657)
  line L531 (110.155, -9.1657) -> (109.9996, -9.2783)
  line L532 (109.9996, -9.2783) -> (109.8263, -9.3931)
  line L533 (109.8263, -9.3931) -> (109.6331, -9.5098)
  line L534 (109.6331, -9.5098) -> (109.4227, -9.6252)
  line L535 (109.4227, -9.6252) -> (109.1918, -9.7395)
  line L536 (109.1918, -9.7395) -> (108.941, -9.8508)
  line L537 (108.941, -9.8508) -> (108.6707, -9.9575)
  line L538 (108.6707, -9.9575) -> (108.4301, -10.0416)
  arc A9 (107.48, -9.3514) -> (108.4301, -10.0416) centre (115, 0.0001) ccw
  line L539 (107.48, -9.3514) -> (107.4857, -9.0966)
  point P0 (107.48, -9.3514)
  point P1 (108.4301, -10.0416)
  point P2 (114.4128, -11.9856)
  point P3 (115.5872, -11.9856)
  point P4 (121.5699, -10.0416)
  point P5 (122.52, -9.3514)
  point P6 (126.2175, -4.2622)
  point P7 (126.5804, -3.1453)
  point P8 (126.5804, 3.1453)
  point P9 (126.2175, 4.2622)
  point P10 (122.52, 9.3514)
  point P11 (121.5699, 10.0416)
  point P12 (115.5872, 11.9856)
  point P13 (114.4128, 11.9856)
  point P14 (108.4301, 10.0416)
  point P15 (107.48, 9.3514)
  point P16 (103.7825, 4.2622)
  point P17 (103.4196, 3.1453)
  point P18 (103.4196, -3.1453)
  point P19 (103.7825, -4.2622)
  constraints: 1080 end point, 20 point on circle, 10 centre point
sketch "layer1" plane through (0, 0, 0) normal (0, 0, 1) x (1, 0, 0)
  line L0 (107.4857, -9.0966) -> (107.5036, -8.8065)
  line L1 (107.5036, -8.8065) -> (107.532, -8.5336)
  line L2 (107.532, -8.5336) -> (107.5694, -8.2786)
  line L3 (107.5694, -8.2786) -> (107.6141, -8.0429)
  line L4 (107.6141, -8.0429) -> (107.6654, -7.8231)
  line L5 (107.6654, -7.8231) -> (107.721, -7.6228)
  line L6 (107.721, -7.6228) -> (107.7801, -7.4403)
  line L7 (107.7801, -7.4403) -> (107.8409, -7.2761)
  line L8 (107.8409, -7.2761) -> (107.9625, -7.0011)
  line L9 (107.9625, -7.0011) -> (108.0758, -6.7937)
  line L10 (108.0758, -6.7937) -> (108.1683, -6.6535)
  line L11 (108.1683, -6.6535) -> (108.218, -6.5889)
  line L12 (108.218, -6.5889) -> (108.3789, -6.4763)
  line L13 (108.3789, -6.4763) -> (108.5412, -6.345)
  line L14 (108.5412, -6.345) -> (108.681, -6.2122)
  line L15 (108.681, -6.2122) -> (108.7986, -6.0795)
  line L16 (108.7986, -6.0795) -> (108.8943, -5.9486)
  line L17 (108.8943, -5.9486) -> (108.9684, -5.821)
  line L18 (108.9684, -5.821) -> (109.0215, -5.6982)
  line L19 (109.0215, -5.6982) -> (109.054, -5.5819)
  line L20 (109.054, -5.5819) -> (109.0667, -5.4735)
  line L21 (109.0667, -5.4735) -> (109.0602, -5.3745)
  line L22 (109.0602, -5.3745) -> (109.0355, -5.2862)
  line L23 (109.0355, -5.2862) -> (108.987, -5.2014)
  line L24 (108.987, -5.2014) -> (108.8344, -5.0188)
  line L25 (108.8344, -5.0188) -> (108.5683, -4.6729)
  line L26 (108.5683, -4.6729) -> (108.3216, -4.313)
  line L27 (108.3216, -4.313) -> (108.1951, -4.1114)
  line L28 (108.1951, -4.1114) -> (108.1294, -4.0391)
  line L29 (108.1294, -4.0391) -> (108.0531, -3.9883)
  line L30 (108.0531, -3.9883) -> (107.9608, -3.9515)
  line L31 (107.9608, -3.9515) -> (107.8538, -3.9301)
  line L32 (107.8538, -3.9301) -> (107.7332, -3.9251)
  line L33 (107.7332, -3.9251) -> (107.6001, -3.9376)
  line L34 (107.6001, -3.9376) -> (107.4558, -3.9687)
  line L35 (107.4558, -3.9687) -> (107.3017, -4.0192)
  line L36 (107.3017, -4.0192) -> (107.1392, -4.0901)
  line L37 (107.1392, -4.0901) -> (106.9697, -4.182)
  line L38 (106.9697, -4.182) -> (106.7947, -4.2958)
  line L39 (106.7947, -4.2958) -> (106.6379, -4.414)
  line L40 (106.6379, -4.414) -> (106.561, -4.4413)
  line L41 (106.561, -4.4413) -> (106.3991, -4.4859)
  line L42 (106.3991, -4.4859) -> (106.1668, -4.5296)
  line L43 (106.1668, -4.5296) -> (105.8678, -4.5603)
  line L44 (105.8678, -4.5603) -> (105.6928, -4.5674)
  line L45 (105.6928, -4.5674) -> (105.5009, -4.5671)
  line L46 (105.5009, -4.5671) -> (105.2933, -4.5582)
  line L47 (105.2933, -4.5582) -> (105.0683, -4.539)
  line L48 (105.0683, -4.539) -> (104.8304, -4.5087)
  line L49 (104.8304, -4.5087) -> (104.5763, -4.4654)
  line L50 (104.5763, -4.4654) -> (104.308, -4.4081)
  line L51 (104.308, -4.4081) -> (104.0266, -4.3355)
  line L52 (104.0266, -4.3355) -> (103.7825, -4.2622)
  arc A0 (103.4196, -3.1453) -> (103.7825, -4.2622) centre (115.0001, 0) ccw
  line L53 (103.4196, -3.1453) -> (103.574, -2.9425)
  line L54 (103.574, -2.9425) -> (103.759, -2.7184)
  line L55 (103.759, -2.7184) -> (103.9423, -2.5143)
  line L56 (103.9423, -2.5143) -> (104.1225, -2.33)
  line L57 (104.1225, -2.33) -> (104.2971, -2.1655)
  line L58 (104.2971, -2.1655) -> (104.4678, -2.0178)
  line L59 (104.4678, -2.0178) -> (104.6306, -1.8885)
  line L60 (104.6306, -1.8885) -> (104.7857, -1.7756)
  line L61 (104.7857, -1.7756) -> (104.9314, -1.6785)
  line L62 (104.9314, -1.6785) -> (105.1914, -1.5275)
  line L63 (105.1914, -1.5275) -> (105.405, -1.4263)
  line L64 (105.405, -1.4263) -> (105.5622, -1.3672)
  line L65 (105.5622, -1.3672) -> (105.6405, -1.3442)
  line L66 (105.6405, -1.3442) -> (105.8368, -1.3476)
  line L67 (105.8368, -1.3476) -> (106.0452, -1.3368)
  line L68 (106.0452, -1.3368) -> (106.2364, -1.3115)
  line L69 (106.2364, -1.3115) -> (106.4095, -1.2733)
  line L70 (106.4095, -1.2733) -> (106.5639, -1.2237)
  line L71 (106.5639, -1.2237) -> (106.6989, -1.164)
  line L72 (106.6989, -1.164) -> (106.8139, -1.0959)
  line L73 (106.8139, -1.0959) -> (106.9086, -1.0209)
  line L74 (106.9086, -1.0209) -> (106.9826, -0.9407)
  line L75 (106.9826, -0.9407) -> (107.0356, -0.8567)
  line L76 (107.0356, -0.8567) -> (107.0675, -0.7708)
  line L77 (107.0675, -0.7708) -> (107.0781, -0.6736)
  line L78 (107.0781, -0.6736) -> (107.062, -0.4362)
  line L79 (107.062, -0.4362) -> (107.05, 0)
  line L80 (107.05, 0) -> (107.062, 0.4362)
  line L81 (107.062, 0.4362) -> (107.0781, 0.6736)
  line L82 (107.0781, 0.6736) -> (107.0675, 0.7708)
  line L83 (107.0675, 0.7708) -> (107.0356, 0.8567)
  line L84 (107.0356, 0.8567) -> (106.9826, 0.9407)
  line L85 (106.9826, 0.9407) -> (106.9086, 1.0209)
  line L86 (106.9086, 1.0209) -> (106.8139, 1.0959)
  line L87 (106.8139, 1.0959) -> (106.6989, 1.164)
  line L88 (106.6989, 1.164) -> (106.5639, 1.2237)
  line L89 (106.5639, 1.2237) -> (106.4095, 1.2733)
  line L90 (106.4095, 1.2733) -> (106.2364, 1.3115)
  line L91 (106.2364, 1.3115) -> (106.0452, 1.3368)
  line L92 (106.0452, 1.3368) -> (105.8368, 1.3476)
  line L93 (105.8368, 1.3476) -> (105.6405, 1.3442)
  line L94 (105.6405, 1.3442) -> (105.5622, 1.3672)
  line L95 (105.5622, 1.3672) -> (105.405, 1.4263)
  line L96 (105.405, 1.4263) -> (105.1914, 1.5275)
  line L97 (105.1914, 1.5275) -> (104.9314, 1.6785)
  line L98 (104.9314, 1.6785) -> (104.7857, 1.7756)
  line L99 (104.7857, 1.7756) -> (104.6306, 1.8885)
  line L100 (104.6306, 1.8885) -> (104.4678, 2.0178)
  line L101 (104.4678, 2.0178) -> (104.2971, 2.1655)
  line L102 (104.2971, 2.1655) -> (104.1225, 2.33)
  line L103 (104.1225, 2.33) -> (103.9423, 2.5143)
  line L104 (103.9423, 2.5143) -> (103.759, 2.7184)
  line L105 (103.759, 2.7184) -> (103.574, 2.9425)
  line L106 (103.574, 2.9425) -> (103.4196, 3.1453)
  arc A1 (103.7825, 4.2622) -> (103.4196, 3.1453) centre (115.0001, 0) ccw
  line L107 (103.7825, 4.2622) -> (104.0266, 4.3355)
  line L108 (104.0266, 4.3355) -> (104.308, 4.4081)
  line L109 (104.308, 4.4081) -> (104.5763, 4.4654)
  line L110 (104.5763, 4.4654) -> (104.8304, 4.5087)
  line L111 (104.8304, 4.5087) -> (105.0683, 4.539)
  line L112 (105.0683, 4.539) -> (105.2933, 4.5582)
  line L113 (105.2933, 4.5582) -> (105.5009, 4.5671)
  line L114 (105.5009, 4.5671) -> (105.6928, 4.5674)
  line L115 (105.6928, 4.5674) -> (105.8678, 4.5603)
  line L116 (105.8678, 4.5603) -> (106.1668, 4.5296)
  line L117 (106.1668, 4.5296) -> (106.3991, 4.4859)
  line L118 (106.3991, 4.4859) -> (106.561, 4.4413)
  line L119 (106.561, 4.4413) -> (106.6379, 4.414)
  line L120 (106.6379, 4.414) -> (106.7947, 4.2958)
  line L121 (106.7947, 4.2958) -> (106.9697, 4.182)
  line L122 (106.9697, 4.182) -> (107.1392, 4.0901)
  line L123 (107.1392, 4.0901) -> (107.3017, 4.0192)
  line L124 (107.3017, 4.0192) -> (107.4558, 3.9687)
  line L125 (107.4558, 3.9687) -> (107.6001, 3.9376)
  line L126 (107.6001, 3.9376) -> (107.7332, 3.9251)
  line L127 (107.7332, 3.9251) -> (107.8538, 3.9301)
  line L128 (107.8538, 3.9301) -> (107.9608, 3.9515)
  line L129 (107.9608, 3.9515) -> (108.0531, 3.9883)
  line L130 (108.0531, 3.9883) -> (108.1294, 4.0391)
  line L131 (108.1294, 4.0391) -> (108.1951, 4.1114)
  line L132 (108.1951, 4.1114) -> (108.3216, 4.313)
  line L133 (108.3216, 4.313) -> (108.5683, 4.6729)
  line L134 (108.5683, 4.6729) -> (108.8344, 5.0188)
  line L135 (108.8344, 5.0188) -> (108.987, 5.2014)
  line L136 (108.987, 5.2014) -> (109.0355, 5.2862)
  line L137 (109.0355, 5.2862) -> (109.0602, 5.3745)
  line L138 (109.0602, 5.3745) -> (109.0667, 5.4735)
  line L139 (109.0667, 5.4735) -> (109.054, 5.5819)
  line L140 (109.054, 5.5819) -> (109.0215, 5.6982)
  line L141 (109.0215, 5.6982) -> (108.9684, 5.821)
  line L142 (108.9684, 5.821) -> (108.8943, 5.9486)
  line L143 (108.8943, 5.9486) -> (108.7986, 6.0795)
  line L144 (108.7986, 6.0795) -> (108.681, 6.2122)
  line L145 (108.681, 6.2122) -> (108.5412, 6.345)
  line L146 (108.5412, 6.345) -> (108.3789, 6.4763)
  line L147 (108.3789, 6.4763) -> (108.218, 6.5889)
  line L148 (108.218, 6.5889) -> (108.1683, 6.6535)
  line L149 (108.1683, 6.6535) -> (108.0758, 6.7937)
  line L150 (108.0758, 6.7937) -> (107.9625, 7.0011)
  line L151 (107.9625, 7.0011) -> (107.8409, 7.2761)
  line L152 (107.8409, 7.2761) -> (107.7801, 7.4403)
  line L153 (107.7801, 7.4403) -> (107.721, 7.6228)
  line L154 (107.721, 7.6228) -> (107.6654, 7.8231)
  line L155 (107.6654, 7.8231) -> (107.6141, 8.0429)
  line L156 (107.6141, 8.0429) -> (107.5694, 8.2786)
  line L157 (107.5694, 8.2786) -> (107.532, 8.5336)
  line L158 (107.532, 8.5336) -> (107.5036, 8.8065)
  line L159 (107.5036, 8.8065) -> (107.4857, 9.0966)
  line L160 (107.4857, 9.0966) -> (107.48, 9.3514)
  arc A2 (108.4301, 10.0416) -> (107.48, 9.3514) centre (115, -0.0001) ccw
  line L161 (108.4301, 10.0416) -> (108.6707, 9.9575)
  line L162 (108.6707, 9.9575) -> (108.941, 9.8508)
  line L163 (108.941, 9.8508) -> (109.1918, 9.7395)
  line L164 (109.1918, 9.7395) -> (109.4227, 9.6252)
  line L165 (109.4227, 9.6252) -> (109.6331, 9.5098)
  line L166 (109.6331, 9.5098) -> (109.8263, 9.3931)
  line L167 (109.8263, 9.3931) -> (109.9996, 9.2783)
  line L168 (109.9996, 9.2783) -> (110.155, 9.1657)
  line L169 (110.155, 9.1657) -> (110.2923, 9.0571)
  line L170 (110.2923, 9.0571) -> (110.5162, 8.8565)
  line L171 (110.5162, 8.8565) -> (110.6785, 8.6847)
  line L172 (110.6785, 8.6847) -> (110.7833, 8.5534)
  line L173 (110.7833, 8.5534) -> (110.8294, 8.4861)
  line L174 (110.8294, 8.4861) -> (110.8867, 8.2983)
  line L175 (110.8867, 8.2983) -> (110.9615, 8.1034)
  line L176 (110.9615, 8.1034) -> (111.0445, 7.9294)
  line L177 (111.0445, 7.9294) -> (111.1344, 7.7765)
  line L178 (111.1344, 7.7765) -> (111.2293, 7.6451)
  line L179 (111.2293, 7.6451) -> (111.3278, 7.5351)
  line L180 (111.3278, 7.5351) -> (111.4281, 7.4468)
  line L181 (111.4281, 7.4468) -> (111.5287, 7.3799)
  line L182 (111.5287, 7.3799) -> (111.6279, 7.3344)
  line L183 (111.6279, 7.3344) -> (111.724, 7.3099)
  line L184 (111.724, 7.3099) -> (111.8157, 7.3061)
  line L185 (111.8157, 7.3061) -> (111.9113, 7.3261)
  line L186 (111.9113, 7.3261) -> (112.1321, 7.4147)
  line L187 (112.1321, 7.4147) -> (112.5433, 7.5609)
  line L188 (112.5433, 7.5609) -> (112.9619, 7.6843)
  line L189 (112.9619, 7.6843) -> (113.1926, 7.7424)
  line L190 (113.1926, 7.7424) -> (113.2818, 7.7825)
  line L191 (113.2818, 7.7825) -> (113.3537, 7.8394)
  line L192 (113.3537, 7.8394) -> (113.4171, 7.9157)
  line L193 (113.4171, 7.9157) -> (113.4706, 8.0109)
  line L194 (113.4706, 8.0109) -> (113.5126, 8.1241)
  line L195 (113.5126, 8.1241) -> (113.5418, 8.2545)
  line L196 (113.5418, 8.2545) -> (113.5569, 8.4013)
  line L197 (113.5569, 8.4013) -> (113.5564, 8.5635)
  line L198 (113.5564, 8.5635) -> (113.5393, 8.74)
  line L199 (113.5393, 8.74) -> (113.5042, 8.9296)
  line L200 (113.5042, 8.9296) -> (113.4501, 9.1312)
  line L201 (113.4501, 9.1312) -> (113.3861, 9.3168)
  line L202 (113.3861, 9.3168) -> (113.3839, 9.3984)
  line L203 (113.3839, 9.3984) -> (113.3915, 9.5662)
  line L204 (113.3915, 9.5662) -> (113.4217, 9.8006)
  line L205 (113.4217, 9.8006) -> (113.485, 10.0945)
  line L206 (113.485, 10.0945) -> (113.5322, 10.2631)
  line L207 (113.5322, 10.2631) -> (113.5918, 10.4455)
  line L208 (113.5918, 10.4455) -> (113.6644, 10.6402)
  line L209 (113.6644, 10.6402) -> (113.7522, 10.8482)
  line L210 (113.7522, 10.8482) -> (113.8546, 11.0652)
  line L211 (113.8546, 11.0652) -> (113.9742, 11.2934)
  line L212 (113.9742, 11.2934) -> (114.1116, 11.5309)
  line L213 (114.1116, 11.5309) -> (114.2676, 11.7761)
  line L214 (114.2676, 11.7761) -> (114.4128, 11.9856)
  arc A3 (115.5872, 11.9856) -> (114.4128, 11.9856) centre (115, -0.0001) ccw
  line L215 (115.5872, 11.9856) -> (115.7324, 11.7761)
  line L216 (115.7324, 11.7761) -> (115.8884, 11.5309)
  line L217 (115.8884, 11.5309) -> (116.0258, 11.2934)
  line L218 (116.0258, 11.2934) -> (116.1454, 11.0652)
  line L219 (116.1454, 11.0652) -> (116.2478, 10.8482)
  line L220 (116.2478, 10.8482) -> (116.3356, 10.6402)
  line L221 (116.3356, 10.6402) -> (116.4082, 10.4455)
  line L222 (116.4082, 10.4455) -> (116.4678, 10.2631)
  line L223 (116.4678, 10.2631) -> (116.515, 10.0945)
  line L224 (116.515, 10.0945) -> (116.5783, 9.8006)
  line L225 (116.5783, 9.8006) -> (116.6085, 9.5662)
  line L226 (116.6085, 9.5662) -> (116.6161, 9.3984)
  line L227 (116.6161, 9.3984) -> (116.6139, 9.3168)
  line L228 (116.6139, 9.3168) -> (116.5499, 9.1312)
  line L229 (116.5499, 9.1312) -> (116.4958, 8.9296)
  line L230 (116.4958, 8.9296) -> (116.4607, 8.74)
  line L231 (116.4607, 8.74) -> (116.4436, 8.5635)
  line L232 (116.4436, 8.5635) -> (116.4431, 8.4013)
  line L233 (116.4431, 8.4013) -> (116.4582, 8.2545)
  line L234 (116.4582, 8.2545) -> (116.4874, 8.1241)
  line L235 (116.4874, 8.1241) -> (116.5294, 8.0109)
  line L236 (116.5294, 8.0109) -> (116.5829, 7.9157)
  line L237 (116.5829, 7.9157) -> (116.6463, 7.8394)
  line L238 (116.6463, 7.8394) -> (116.7182, 7.7825)
  line L239 (116.7182, 7.7825) -> (116.8074, 7.7424)
  line L240 (116.8074, 7.7424) -> (117.0381, 7.6843)
  line L241 (117.0381, 7.6843) -> (117.4567, 7.5609)
  line L242 (117.4567, 7.5609) -> (117.8679, 7.4147)
  line L243 (117.8679, 7.4147) -> (118.0887, 7.3261)
  line L244 (118.0887, 7.3261) -> (118.1843, 7.3061)
  line L245 (118.1843, 7.3061) -> (118.276, 7.3099)
  line L246 (118.276, 7.3099) -> (118.3721, 7.3344)
  line L247 (118.3721, 7.3344) -> (118.4713, 7.3799)
  line L248 (118.4713, 7.3799) -> (118.5719, 7.4468)
  line L249 (118.5719, 7.4468) -> (118.6722, 7.5351)
  line L250 (118.6722, 7.5351) -> (118.7707, 7.6451)
  line L251 (118.7707, 7.6451) -> (118.8656, 7.7765)
  line L252 (118.8656, 7.7765) -> (118.9555, 7.9294)
  line L253 (118.9555, 7.9294) -> (119.0385, 8.1034)
  line L254 (119.0385, 8.1034) -> (119.1133, 8.2983)
  line L255 (119.1133, 8.2983) -> (119.1706, 8.4861)
  line L256 (119.1706, 8.4861) -> (119.2167, 8.5534)
  line L257 (119.2167, 8.5534) -> (119.3215, 8.6847)
  line L258 (119.3215, 8.6847) -> (119.4838, 8.8565)
  line L259 (119.4838, 8.8565) -> (119.7077, 9.0571)
  line L260 (119.7077, 9.0571) -> (119.845, 9.1657)
  line L261 (119.845, 9.1657) -> (120.0004, 9.2783)
  line L262 (120.0004, 9.2783) -> (120.1737, 9.3931)
  line L263 (120.1737, 9.3931) -> (120.3669, 9.5098)
  line L264 (120.3669, 9.5098) -> (120.5773, 9.6252)
  line L265 (120.5773, 9.6252) -> (120.8082, 9.7395)
  line L266 (120.8082, 9.7395) -> (121.059, 9.8508)
  line L267 (121.059, 9.8508) -> (121.3293, 9.9575)
  line L268 (121.3293, 9.9575) -> (121.5699, 10.0416)
  arc A4 (122.52, 9.3514) -> (121.5699, 10.0416) centre (115, -0.0001) ccw
  line L269 (122.52, 9.3514) -> (122.5143, 9.0966)
  line L270 (122.5143, 9.0966) -> (122.4964, 8.8065)
  line L271 (122.4964, 8.8065) -> (122.468, 8.5336)
  line L272 (122.468, 8.5336) -> (122.4306, 8.2786)
  line L273 (122.4306, 8.2786) -> (122.3859, 8.0429)
  line L274 (122.3859, 8.0429) -> (122.3346, 7.8231)
  line L275 (122.3346, 7.8231) -> (122.279, 7.6228)
  line L276 (122.279, 7.6228) -> (122.2199, 7.4403)
  line L277 (122.2199, 7.4403) -> (122.1591, 7.2761)
  line L278 (122.1591, 7.2761) -> (122.0375, 7.0011)
  line L279 (122.0375, 7.0011) -> (121.9242, 6.7937)
  line L280 (121.9242, 6.7937) -> (121.8317, 6.6535)
  line L281 (121.8317, 6.6535) -> (121.782, 6.5889)
  line L282 (121.782, 6.5889) -> (121.6211, 6.4763)
  line L283 (121.6211, 6.4763) -> (121.4588, 6.345)
  line L284 (121.4588, 6.345) -> (121.319, 6.2122)
  line L285 (121.319, 6.2122) -> (121.2014, 6.0795)
  line L286 (121.2014, 6.0795) -> (121.1057, 5.9486)
  line L287 (121.1057, 5.9486) -> (121.0316, 5.821)
  line L288 (121.0316, 5.821) -> (120.9785, 5.6982)
  line L289 (120.9785, 5.6982) -> (120.946, 5.5819)
  line L290 (120.946, 5.5819) -> (120.9333, 5.4735)
  line L291 (120.9333, 5.4735) -> (120.9398, 5.3745)
  line L292 (120.9398, 5.3745) -> (120.9645, 5.2862)
  line L293 (120.9645, 5.2862) -> (121.013, 5.2014)
  line L294 (121.013, 5.2014) -> (121.1656, 5.0188)
  line L295 (121.1656, 5.0188) -> (121.4317, 4.6729)
  line L296 (121.4317, 4.6729) -> (121.6784, 4.313)
  line L297 (121.6784, 4.313) -> (121.8049, 4.1114)
  line L298 (121.8049, 4.1114) -> (121.8706, 4.0391)
  line L299 (121.8706, 4.0391) -> (121.9469, 3.9883)
  line L300 (121.9469, 3.9883) -> (122.0392, 3.9515)
  line L301 (122.0392, 3.9515) -> (122.1462, 3.9301)
  line L302 (122.1462, 3.9301) -> (122.2668, 3.9251)
  line L303 (122.2668, 3.9251) -> (122.3999, 3.9376)
  line L304 (122.3999, 3.9376) -> (122.5442, 3.9687)
  line L305 (122.5442, 3.9687) -> (122.6983, 4.0192)
  line L306 (122.6983, 4.0192) -> (122.8608, 4.0901)
  line L307 (122.8608, 4.0901) -> (123.0303, 4.182)
  line L308 (123.0303, 4.182) -> (123.2053, 4.2958)
  line L309 (123.2053, 4.2958) -> (123.3621, 4.414)
  line L310 (123.3621, 4.414) -> (123.439, 4.4413)
  line L311 (123.439, 4.4413) -> (123.6009, 4.4859)
  line L312 (123.6009, 4.4859) -> (123.8332, 4.5296)
  line L313 (123.8332, 4.5296) -> (124.1322, 4.5603)
  line L314 (124.1322, 4.5603) -> (124.3072, 4.5674)
  line L315 (124.3072, 4.5674) -> (124.4991, 4.5671)
  line L316 (124.4991, 4.5671) -> (124.7067, 4.5582)
  line L317 (124.7067, 4.5582) -> (124.9317, 4.539)
  line L318 (124.9317, 4.539) -> (125.1696, 4.5087)
  line L319 (125.1696, 4.5087) -> (125.4237, 4.4654)
  line L320 (125.4237, 4.4654) -> (125.692, 4.4081)
  line L321 (125.692, 4.4081) -> (125.9734, 4.3355)
  line L322 (125.9734, 4.3355) -> (126.2175, 4.2622)
  arc A5 (126.5804, 3.1453) -> (126.2175, 4.2622) centre (114.9999, 0) ccw
  line L323 (126.5804, 3.1453) -> (126.426, 2.9425)
  line L324 (126.426, 2.9425) -> (126.241, 2.7184)
  line L325 (126.241, 2.7184) -> (126.0577, 2.5143)
  line L326 (126.0577, 2.5143) -> (125.8775, 2.33)
  line L327 (125.8775, 2.33) -> (125.7029, 2.1655)
  line L328 (125.7029, 2.1655) -> (125.5322, 2.0178)
  line L329 (125.5322, 2.0178) -> (125.3694, 1.8885)
  line L330 (125.3694, 1.8885) -> (125.2143, 1.7756)
  line L331 (125.2143, 1.7756) -> (125.0686, 1.6785)
  line L332 (125.0686, 1.6785) -> (124.8086, 1.5275)
  line L333 (124.8086, 1.5275) -> (124.595, 1.4263)
  line L334 (124.595, 1.4263) -> (124.4378, 1.3672)